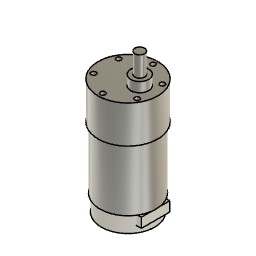
MG540直流减速电机（GMR） v8 (Autodesk Fusion 360 design; units mm, degrees)
Autodesk Fusion 360 part; units mm, degrees
sketch "草图1" plane through (0, 0, 0) normal (0, 0, 1) x (1, 0, 0)
  circle A0 centre (0, 0) radius 16.375
  dimension "d1" = 32.75
  constraint coincident A0.centre origin
  measures "d1" diameter of A0
extrude "拉伸1" add sketch "草图1" along normal blind 10.05 makes body 1
sketch "草图3" plane through (0, 0, 10.05) normal (0, 0, 1) x (-1, 0, 0)
  circle A0 centre (0, 0) radius 16.375
  line L0 (5, 0) -> (-14, 0)
  line L1 (-10, -8.75) -> (-17, -8.75)
  line L2 (-17, -8.75) -> (-17, 8.75)
  line L3 (-17, 8.75) -> (-10, 8.75)
  line L4 (-10, 8.75) -> (-10, -8.75)
  dimension "d5" = 17.5
  dimension "d6" = 7
  dimension "d7" = 10
  constraint horizontal L0
  constraint horizontal L1
  constraint vertical L2
  constraint horizontal L3
  constraint vertical L4
  constraint symmetric L0 L1 L3
  constraint coincident A0.centre L0
  measures "d5" distance of L1.start L3.end
  measures "d6" distance of L1.start L1.end
  measures "d7" distance of A0.centre L4
extrude "拉伸2" add sketch "草图3" against normal blind 6 separate body contours A0 L1 L3 L4 | A0 L1 L2 L3 picked at (-11.6443, -5.1563) makes body 2
sketch "草图4" plane through (0, 0, 10.05) normal (0, 0, 1) x (-1, 0, 0)
  circle A0 centre (0, 0) radius 16.375
  circle A1 centre (0, 0) radius 17.2
  dimension "d10" = 34.4
  constraint coincident A0.centre A1.centre
  measures "d10" diameter of A1
extrude "拉伸3" add sketch "草图4" along normal blind 38 separate body contours A0 | A1 makes body 3
sketch "草图5" plane through (0, 0, 48.05) normal (0, 0, 1) x (-1, 0, 0)
  circle A0 centre (0, 0) radius 17.2
  circle A1 centre (0, 0) radius 18.35
  dimension "d13" = 36.7
  constraint coincident A0.centre A1.centre
  measures "d13" diameter of A1
extrude "拉伸4" add sketch "草图5" along normal blind 23 separate body contours A0 | A1 makes body 4
sketch "草图6" plane through (0, 0, 71.05) normal (0, 0, 1) x (-1, 0, 0)
  circle A0 centre (0, 0) radius 18.35
  circle A1 centre (0, 0) radius 15.5 construction
  circle A2 centre (0, 15.5) radius 1.5
  line L0 (0, -7) -> (0, 24)
  circle A3 centre (-13.4234, 7.75) radius 1.5
  circle A4 centre (-13.4234, -7.75) radius 1.5
  circle A5 centre (0, -15.5) radius 1.5
  circle A6 centre (13.4234, -7.75) radius 1.5
  circle A7 centre (13.4234, 7.75) radius 1.5
  dimension "d16" = 31
  dimension "d17" = 3
  dimension "d19" = 360
  constraint coincident A0.centre A1.centre
  constraint coincident A1 A2.centre
  constraint vertical L0
  constraint coincident A2.centre L0
  constraint coincident A0.centre L0
  measures "d16" diameter of A1
  measures "d17" diameter of A2
extrude "拉伸5" cut sketch "草图6" against normal blind 6 contours A2 L0 | A2 L0 | A3 | A4 | A5 | A6 | A7 bodies 4
sketch "草图7" plane through (0, 0, 71.05) normal (0, 0, 1) x (-1, 0, 0)
  circle A0 centre (-13.4234, -7.75) radius 1.5
  circle A1 centre (-13.4234, 7.75) radius 1.5
  circle A2 centre (0, -15.5) radius 1.5
  circle A3 centre (13.4234, 7.75) radius 1.5
  circle A4 centre (0, 15.5) radius 1.5
  circle A5 centre (13.4234, -7.75) radius 1.5
  circle A6 centre (0, 0) radius 18.35
  circle A7 centre (-7.25, 0) radius 5.5
  dimension "d22" = 11
  dimension "d23" = 7.25
  measures "d22" diameter of A7
  measures "d23" distance of A6.centre A7.centre
extrude "拉伸6" add sketch "草图7" along normal blind 6 separate body contours A7 makes body 5
sketch "草图8" plane through (0, 0, 77.05) normal (0, 0, 1) x (-1, 0, 0)
  circle A0 centre (-7.25, 0) radius 5.5
  circle A1 centre (-7.25, 0) radius 3
  dimension "d26" = 6
  constraint concentric A0 A1
  measures "d26" diameter of A1
extrude "拉伸7" add sketch "草图8" along normal blind 12.45 separate body contours A1 makes body 6
copy_body "实体->零部件1" bodies 1 removing the originals makes body 7 in component "GMR编码器"
copy_body "实体->零部件2" bodies 2 removing the originals makes body 8 in component "6p pin"
copy_body "实体->零部件3" bodies 3 removing the originals makes body 9 in component "电机"
copy_body "实体->零部件4" bodies 4 removing the originals makes body 10 in component "减速箱"
copy_body "实体->零部件5" bodies 5 removing the originals makes body 11 in component "Component''''"
copy_body "实体->零部件6" bodies 6 removing the originals makes body 12 in component "输出轴"
component "GMR编码器" placed x (1, 0, 0) y (0, 1, 0) z (0, 0, 1) at (0, 0, 0)
component "6p pin" placed x (1, 0, 0) y (0, 1, 0) z (0, 0, 1) at (0, 0, 0)
component "电机" placed x (1, 0, 0) y (0, 1, 0) z (0, 0, 1) at (0, 0, 0)
component "减速箱" placed x (1, 0, 0) y (0, 1, 0) z (0, 0, 1) at (0, 0, 0)
component "Component''''" placed x (1, 0, 0) y (0, 1, 0) z (0, 0, 1) at (0, 0, 0)
component "输出轴" placed x (1, 0, 0) y (0, 1, 0) z (0, 0, 1) at (0, 0, 0)
named bodies: "GMR编码器", "6p pin", "电机", "减速箱", "输出轴"
